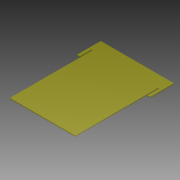
# Autodesk Inventor part: door
Saved by Autodesk Inventor 2014 SP2 (Build 180246200, 246)
## iProperties
Created: 2016-05-06
Part Number: door
Material: Generic
Document SubType Name: Modeling
Designer: cruiser
Density: 1 g/cm^3
Appearance: Clear - Yellow
Author: cruiser
Autodesk Inventor part; units mm, degrees
ref_plane "YZ Plane" through (0, 0, 0) normal (1, 0, 0) x (0, 1, 0)
ref_plane "XZ Plane" through (0, 0, 0) normal (0, 1, 0) x (-1, 0, 0)
ref_plane "XY Plane" through (0, 0, 0) normal (0, 0, 1) x (1, 0, 0)
sketch "Sketch1" plane through (0, 0, 0) normal (0, 0, 1) x (1, 0, 0)
  line L0 (110.5, -144.9563) -> (-110.5, -144.9563)
  line L1 (-110.5, -144.9563) -> (-110.5, 144.9562)
  line L2 (-110.5, 144.9562) -> (110.5, 144.9563)
  line L3 (110.5, 144.9563) -> (110.5, -144.9563)
  line L4 (110.5, -144.9563) -> (-110.5, 144.9562) construction
  line L5 (-110.5, -144.9563) -> (110.5, 144.9563) construction
  line L6 (-110.5, -144.9563) -> (110.5, -144.9563)
  line L7 (110.5, -144.9563) -> (110.5, -174.9563)
  line L8 (110.5, -174.9563) -> (-110.5, -174.9563)
  line L9 (-110.5, -174.9563) -> (-110.5, -144.9563)
  point P0 (0, 0)
  dimension "d0" = 221
  dimension "d1" = 289.9125
  dimension "d4" = 30
  dimension "d5" = 0
  dimension "d6" = 0
  constraints: 20 end point, 4 parallel, 2 horizontal, 2 midpoint, 2 perpendicular, 1 point on line
  measures "d0" distance of L1.end L2.end
  measures "d1" distance of L0.end L1.end
  measures "d4" distance of L6.end L7.end
  measures "d5" distance between parallel lines of L1 L9
  measures "d6" distance between parallel lines of L3 L7
extrude "Extrusion1" add sketch "Sketch1" along normal blind 3.15
sketch "Sketch2" plane through (0, 0, 3.15) normal (0, 0, 1) x (1, 0, 0)
  line L0 (110.5, 144.9563) -> (-110.5, 144.9562) projected
  line L1 (-110.5, 144.9562) -> (-123.65, 144.9562)
  line L2 (-123.65, 144.9562) -> (-123.65, 64.9562)
  line L3 (-123.65, 64.9562) -> (-110.5, 64.9562)
  line L4 (-110.5, 64.9562) -> (-110.5, 144.9562)
  line L5 (-110.5, 64.9562) -> (-113.65, 64.9562)
  line L6 (-113.65, 64.9562) -> (-113.65, 104.9562)
  line L7 (-113.65, 104.9562) -> (-110.5, 104.9562)
  line L8 (-110.5, 104.9562) -> (-110.5, 64.9562)
  line L9 (0, 144.9563) -> (0, 0)
  line L10 (110.5, 144.9563) -> (123.65, 144.9562)
  line L11 (123.65, 144.9562) -> (123.65, 64.9562)
  line L12 (123.65, 64.9562) -> (110.5, 64.9562)
  line L13 (110.5, 64.9562) -> (110.5, 144.9563)
  line L14 (110.5, 64.9562) -> (113.65, 64.9562)
  line L15 (113.65, 64.9562) -> (113.65, 104.9562)
  line L16 (113.65, 104.9562) -> (110.5, 104.9562)
  line L17 (110.5, 104.9562) -> (110.5, 64.9562)
  dimension "d7" = 80
  dimension "d8" = 13.15
  dimension "d9" = 3.15
  dimension "d10" = 40
  constraints: 34 end point, 6 symmetric about line, 5 parallel, 2 horizontal, 2 perpendicular, 1 midpoint
  measures "d7" distance of L1.end L2.end
  measures "d8" distance of L0.end L1.end
  measures "d9" distance of L6.end L7.end
  measures "d10" distance between parallel lines of L1 L7
extrude "Extrusion2" add sketch "Sketch2" against normal blind 3.15 contours L4 L7 L6 L3 L2 L1 | L10 L11 L12 L15 L16 L13
equation "\"d0\" = door_x"
equation "\"d1\" = door_z"
equation "\"d4\" = door_overlap"
equation "\"d2\" = clear_acrylic"
equation "\"d7\" = protection_slot_length"
equation "\"d8\" = protection_slot_width + clear_acrylic"
equation "\"d9\" = clear_acrylic"
equation "\"d10\" = 0.5 * protection_slot_length"
equation "\"d11\" = clear_acrylic"
equation "\"sm_thickness\" = 1.5875"
equation "\"very_thick_acrylic\" = 9.45"
equation "\"thick_acrylic\" = 5.88"
equation "\"thin_acrylic\" = 3.15"
equation "\"clear_acrylic\" = 3.15"
equation "\"wood_thickness\" = 6.72"
equation "\"m3_diameter\" = 3.15"
equation "\"m4_diameter\" = 4.2"
equation "\"m5_diameter\" = 5.25"
equation "\"brass_insert_drill\" = 4"
equation "\"m5_brass_insert_drill\" = 6.7"
equation "\"m3_main_length\" = 14"
equation "\"m3_main_nut_width\" = 5.7"
equation "\"m3_main_nut_thickness\" = 2.5"
equation "\"m3_main_extra\" = 1"
equation "\"stepper_screw_space\" = 35"
equation "\"stepper_shaft_diameter\" = 5"
equation "\"stepper_body_diameter\" = 28"
equation "\"laser_body_diameter\" = 12"
equation "\"carrier_y\" = 221"
equation "\"carrier_z\" = 12"
equation "\"visor_x\" = 227.3"
equation "\"visor_y\" = 90.5"
equation "\"protection_slot\" = 44.2"
equation "\"protection_slot_offset\" = 55.25"
equation "\"protection_slot_length\" = 80"
equation "\"window_z\" = 289.9125"
equation "\"window_y\" = 77.0625"
equation "\"door_x\" = 221"
equation "\"door_z\" = 289.9125"
equation "\"door_sensor\" = 35"
equation "\"reservoir_x\" = 181"
equation "\"reservoir_y\" = 181"
equation "\"linear_bearing_spacing\" = 247"
equation "\"threaded_rod_z\" = 203.2"
equation "\"motor_spacing\" = 327"
equation "\"tray_x\" = 221"
equation "\"tray_y\" = 221"
equation "\"bed_x\" = 141"
equation "\"bed_y\" = 141"
equation "\"bed_z\" = 25.4"
equation "\"bed_z2\" = 74.6"
equation "\"crane_z\" = 45"
equation "\"crane_z2\" = 12"
equation "\"end_stop_offset_x\" = 47"
equation "\"end_stop_spacing\" = 19"
equation "\"door_overlap\" = 30"
equation "\"acrylic_into_frame\" = 5"
equation "\"protection_slot_width\" = 10"
equation "\"frame_top_z\" = 336"
equation "\"nema17_x\" = 43"
equation "\"drawer_z_from_bottom\" = 25"
equation "\"laser_diameter\" = 12"
equation "\"t_galvo_frame\" = 6.72"
equation "\"laser_z\" = 18"
equation "\"drawer_y\" = 73.65"
equation "\"laser_y\" = 35"
equation "\"subframe_x\" = 175"
equation "\"galvo_frame_z\" = 65"
equation "\"subframe_y_offset\" = 27.5"
equation "\"drawer_x\" = 227.3"
equation "\"printer_z\" = 289"
equation "\"lcd_x\" = 72"
equation "\"frame_tilt\" = 1deg"
equation "\"frame_foot_z\" = 12"
equation "\"frame_border\" = 41.35"
equation "\"frame_bottom_z\" = 275"
equation "\"z_min_from_center\" = 95"
equation "\"thumb_nut_diameter\" = 7"
equation "\"laser_z_offset\" = 55"
equation "\"laser_y_offset\" = 19.4"
equation "\"thumb_nut_offset_y\" = 0"
equation "\"galvo_frame_y_offset\" = 27.5"
equation "\"frame_total_z\" = 611"
equation "\"galvo_frame_x\" = 66"
equation "\"drawer_z\" = 236.825"
equation "\"laser_x\" = 24"
equation "\"lcd_y\" = 25"
body "Solid1"
